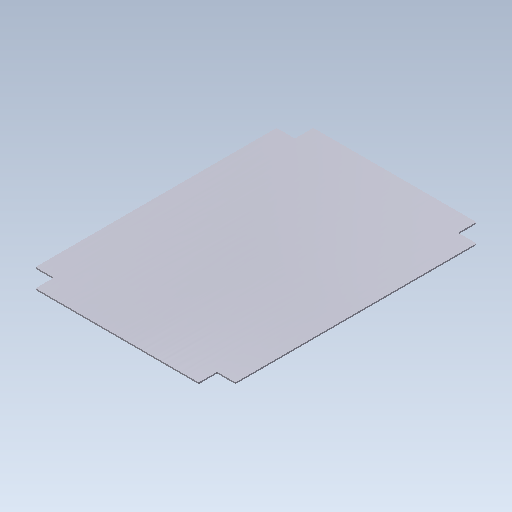
# Autodesk Inventor part: Standard
Saved by Autodesk Inventor 2020.3 (Build 243373000, 373)
## iProperties
RuleStatus: InUse
AfterDocSave0: file://Part Number Cleaner
Created: 2022-01-20
Material: Generic
Catalog Web Link: https://www.janelia.org/
Vendor: HHMI: JRC - jET
Document SubType Name: Modeling
Designer: solomone
Density: 1 g/cm^3
Appearance: Default
LAB/DEPT: A. LEE (LAB)
DESIGN DEPARTMENT: HHMI: JRC - jET
ALTERED ITEM PART NUMBER: N/A
ALTERED ITEM VENDOR: N/A
ALTERED ITEM DESCRIPTION: N/A
Title: Standard
Author: solomone
Revision Number: 0
Autodesk Inventor part; units mm, degrees
ref_plane "YZ Plane" through (0, 0, 0) normal (1, 0, 0) x (0, 1, 0)
ref_plane "XZ Plane" through (0, 0, 0) normal (0, 1, 0) x (-1, 0, 0)
ref_plane "XY Plane" through (0, 0, 0) normal (0, 0, 1) x (1, 0, 0)
sketch "Sketch1" plane through (0, 0, 0) normal (0, 1, 0) x (-1, 0, 0)
  line L0 (186.6, -317.5) -> (-186.6, -317.5)
  line L1 (-228.6, -275.5) -> (-228.6, 275.5)
  line L2 (-186.6, 317.5) -> (186.6, 317.5)
  line L3 (228.6, 275.5) -> (228.6, -275.5)
  line L4 (186.6, -317.5) -> (186.6, -275.5)
  line L5 (186.6, -275.5) -> (228.6, -275.5)
  line L6 (-186.6, -317.5) -> (-186.6, -275.5)
  line L7 (-186.6, -275.5) -> (-228.6, -275.5)
  line L8 (186.6, 317.5) -> (186.6, 275.5)
  line L9 (186.6, 275.5) -> (228.6, 275.5)
  line L10 (-186.6, 317.5) -> (-186.6, 275.5)
  line L11 (-186.6, 275.5) -> (-228.6, 275.5)
  point P0 (0, 0)
  dimension "d5" = 457.2
  dimension "d6" = 228.6
  dimension "d7" = 635
  dimension "d8" = 317.5
  dimension "d9" = 42
  constraints: 24 end point, 7 equal length, 5 horizontal, 2 parallel, 2 point on line, 2 vertical, 1 perpendicular
  measures "d5" distance between parallel lines of L1 L3
  measures "d6" distance from line of point (0, 0) L3
  measures "d7" distance between parallel lines of L2 L0
  measures "d8" distance from line of point (0, 0) L0
  measures "d9" distance of L4.end L3.end
extrude "Extrusion1" add sketch "Sketch1" along normal blind 3.175
fillet "Fillet1" radius 3.175 12 edges at (186.6, 1.5875, -317.5) (186.6, 1.5875, -275.5) (228.6, 1.5875, -275.5) (-186.6, 1.5875, -317.5) (-186.6, 1.5875, -275.5) (-228.6, 1.5875, -275.5) (-228.6, 1.5875, 275.5) (-186.6, 1.5875, 275.5) (-186.6, 1.5875, 317.5) (186.6, 1.5875, 317.5) (186.6, 1.5875, 275.5) (228.6, 1.5875, 275.5)
equation "\"d6\" = 0.5 * d5"
equation "\"d8\" = 0.5 * d7"
body "Solid1"
